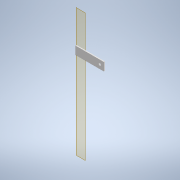
# Autodesk Inventor part: 2x1 Sprocket mount
Saved by Autodesk Inventor 2021 (Build 250183000, 183)
## iProperties
Created: 2021-04-08
Part Number: 2x1 Sprocket mount
Material: Generic
Document SubType Name: Modeling
Designer: con_c_000
Density: 1 g/cm^3
Appearance: Default
Author: con_c_000
Autodesk Inventor part; units mm, degrees
ref_plane "YZ Plane" through (0, 0, 0) normal (1, 0, 0) x (0, 1, 0)
ref_plane "XZ Plane" through (0, 0, 0) normal (0, 1, 0) x (-1, 0, 0)
ref_plane "XY Plane" through (0, 0, 0) normal (0, 0, 1) x (1, 0, 0)
ref_plane "Work Plane1" through (2.1462, -16.6124, 0) normal (0, 0, 1) x (1, 0, 0)
sketch "Sketch1" plane through (2.1462, -16.6124, 0) normal (0, 0, 1) x (1, 0, 0)
  line L0 (-1.0731, 506.7194) -> (165.7814, 506.7194)
  line L1 (165.7814, 506.7194) -> (165.7814, 455.9194)
  line L2 (165.7814, 455.9194) -> (-1.0731, 455.9194)
  line L3 (-1.0731, 455.9194) -> (-1.0731, 506.7194)
  line L4 (24.2028, 585.927) -> (140.3814, 481.3194)
  circle A0 centre (140.3814, 481.3194) radius 6.35
  circle A1 centre (24.2028, 585.927) radius 2.55
  line L5 (-596.0927, 591.4102) -> (-29.8163, 81.5327)
  point P0 (-2.1462, 16.6124)
  dimension "d0" = 50.8
  dimension "d1" = 12.7
  dimension "d2" = 25.4
  dimension "d3" = 25.4
  constraints: 12 end point, 3 parallel, 2 centre point, 2 coincident, 1 horizontal, 1 perpendicular, 2 other
  measures "d0" distance of L0.end L1.end
  measures "d1" diameter of A0
  measures "d2" distance from line of L1 L4.end
  measures "d3" distance from line of L2 L4.end
extrude "Extrusion1" add sketch "Sketch1" along normal blind 6.35 contours L0 L1 L2 L3
body "Solid1"
